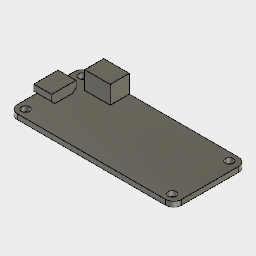
2829 Adafruit Feather Bluefruit 32u4 (Autodesk Fusion 360 design; units mm, degrees)
Autodesk Fusion 360 part; units mm, degrees
sketch "pcb" plane through (0, 0, 0) normal (0, 0, 1) x (1, 0, 0)
  line L0 (0, 0) -> (51.2, 0)
  line L1 (51.2, 0) -> (51.2, 22.8)
  line L2 (51.2, 22.8) -> (0, 22.8)
  line L3 (0, 22.8) -> (0, 0)
  circle A0 centre (2.54, 2.54) radius 1.25
  circle A1 centre (2.54, 20.32) radius 1.25
  circle A2 centre (48.26, 20.32) radius 1.25
  circle A3 centre (48.26, 2.54) radius 1.25
  dimension "d1" = 51.2
  dimension "d2" = 22.8
  dimension "d3" = 2.5
  dimension "d4" = 2.54
  dimension "d5" = 2.54
  dimension "d6" = 2.5
  dimension "d7" = 2.54
  dimension "d8" = 20.32
  dimension "d9" = 2.5
  dimension "d10" = 48.26
  dimension "d11" = 20.32
  dimension "d12" = 2.5
  dimension "d13" = 2.54
  dimension "d14" = 48.26
  measures "d1" distance of L1.end L2.end
  measures "d2" distance of L0.end L1.end
  measures "d3" diameter of A0
  measures "d4" distance of L3 A0.centre
  measures "d5" distance of L0 A0.centre
  measures "d6" diameter of A1
  measures "d7" distance of L3 A1.centre
  measures "d8" distance of L0 A1.centre
  measures "d9" diameter of A2
  measures "d10" distance of L3 A2.centre
  measures "d11" distance of L0 A2.centre
  measures "d12" diameter of A3
  measures "d13" distance of L0 A3.centre
  measures "d14" distance of L3 A3.centre
extrude "Extrude1" add sketch "pcb" against normal blind 1.6 makes body 1
fillet "Fillet1" radius 2.54 4 edges at (0, 0, -0.8) (0, 22.8, -0.8) (51.2, 0, -0.8) (51.2, 22.8, -0.8) on bodies 1
sketch "microusb" plane through (0, 0, 0) normal (0, 0, 1) x (-1, 0, 0)
  arc A0 (-51.2, -20.26) -> (-48.66, -22.8) centre (-48.66, -20.26) ccw
  line L0 (-48.66, -22.8) -> (-2.54, -22.8)
  arc A1 (-2.54, -22.8) -> (0, -20.26) centre (-2.54, -20.26) ccw
  line L1 (0, -20.26) -> (0, -2.54)
  arc A2 (0, -2.54) -> (-2.54, 0) centre (-2.54, -2.54) ccw
  line L2 (-2.54, 0) -> (-48.66, 0)
  arc A3 (-48.66, 0) -> (-51.2, -2.54) centre (-48.66, -2.54) ccw
  line L3 (-51.2, -2.54) -> (-51.2, -20.26)
  circle A4 centre (-2.54, -2.54) radius 1.25
  circle A5 centre (-48.26, -20.32) radius 1.25
  circle A6 centre (-48.26, -2.54) radius 1.25
  circle A7 centre (-2.54, -20.32) radius 1.25
  line L4 (0, -15.23) -> (-5.6, -15.23)
  line L5 (-5.6, -15.23) -> (-5.6, -7.63)
  line L6 (-5.6, -7.63) -> (0, -7.63)
  line L7 (0, -7.63) -> (0, -15.23)
  line L8 (-5.6, -11.43) -> (0, -11.43) construction
  dimension "d18" = 7.6
  dimension "d19" = 5.6
  dimension "d20" = 11.43
  measures "d18" distance of L4.end L5.end
  measures "d19" distance of L4.start L4.end
  measures "d20" distance of L2 L8
extrude "Extrude2" add sketch "microusb" along normal blind 2.95 separate body contours L1 L4 L5 L6 L7 makes body 2
chamfer "Chamfer1" distance 1 angle 45 2 edges at (2.8, 15.23, 0) (2.8, 7.63, 0) on bodies 2
sketch "jst" plane through (0, 0, 0) normal (0, 0, 1) x (-1, 0, 0)
  arc A0 (-51.2, -20.26) -> (-48.66, -22.8) centre (-48.66, -20.26) ccw
  line L0 (-48.66, -22.8) -> (-2.54, -22.8)
  arc A1 (-2.54, -22.8) -> (0, -20.26) centre (-2.54, -20.26) ccw
  line L1 (0, -20.26) -> (0, -2.54)
  arc A2 (0, -2.54) -> (-2.54, 0) centre (-2.54, -2.54) ccw
  line L2 (-2.54, 0) -> (-48.66, 0)
  arc A3 (-48.66, 0) -> (-51.2, -2.54) centre (-48.66, -2.54) ccw
  line L3 (-51.2, -2.54) -> (-51.2, -20.26)
  circle A4 centre (-2.54, -2.54) radius 1.25
  circle A5 centre (-48.26, -20.32) radius 1.25
  circle A6 centre (-48.26, -2.54) radius 1.25
  circle A7 centre (-2.54, -20.32) radius 1.25
  line L4 (-6.668, -22.8) -> (-14.668, -22.8)
  line L5 (-14.668, -22.8) -> (-14.668, -16.8)
  line L6 (-14.668, -16.8) -> (-6.668, -16.8)
  line L7 (-6.668, -16.8) -> (-6.668, -22.8)
  line L8 (-10.668, -22.8) -> (-10.668, -16.8) construction
  dimension "d24" = 8
  dimension "d25" = 6
  dimension "d26" = 10.668
  measures "d24" distance of L4.start L4.end
  measures "d25" distance of L4.start L6.end
  measures "d26" distance of L1 L8
extrude "Extrude3" add sketch "jst" along normal blind 5.6 separate body contours L0 L4 L5 L6 L7 makes body 3
named bodies: "pcb", "usb", "jst"
